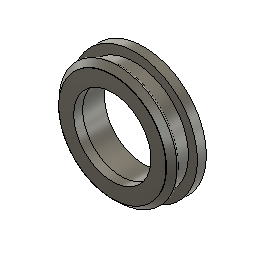
MT2 to 25mm hole sleeve v1 (Autodesk Fusion 360 design; units mm, degrees)
Autodesk Fusion 360 part; units mm, degrees
sketch "Sketch1" plane through (0, 0, 0) normal (0, 0, 1) x (1, 0, 0)
  circle A0 centre (0, 0) radius 8.75
  circle A1 centre (0, 0) radius 12
  circle A2 centre (0, 0) radius 14
  circle A3 centre (0, 0) radius 6
  circle A4 centre (0, 0) radius 2.5
  dimension "d1" = 17.5
  dimension "d2" = 24
  dimension "d3" = 28
  dimension "d8" = 12
  dimension "d11" = 5
  constraint coincident A0.centre A1.centre
  constraint concentric A0 A1
  measures "d1" diameter of A0
  measures "d2" diameter of A1
  measures "d3" diameter of A2
  measures "d8" diameter of A3
  measures "d11" diameter of A4
extrude "Extrude1" add sketch "Sketch1" along normal blind 2 contours A2
extrude "Extrude2" add sketch "Sketch1" along normal blind 5 contours A0 | A1
extrude "Extrude3" cut sketch "Sketch1" along normal blind 5 draft -1.42 contours A0 | A3
sketch "Sketch2" plane through (0, 0, 5) normal (0, 0, 1) x (1, 0, 0)
  circle A0 centre (0, 0) radius 8.6261
  circle A1 centre (0, 0) radius 12
  circle A2 centre (0, 0) radius 8.6261
  circle A3 centre (0, 0) radius 12
  circle A4 centre (0, 0) radius 14
  dimension "d12" = 28
  constraint coincident A0.centre A1.centre
  measures "d12" diameter of A4
extrude "Extrude4" add sketch "Sketch2" along normal blind 2 contours A1 A3
sketch "Sketch3" plane through (0, 0, 0) normal (1, 0, 0) x (0, 0, -1)
  line L0 (-5.3, 12) -> (-5.3, 13)
  line L1 (-5.7268, 13.1768) -> (-6.9036, 12)
  line L2 (-6.9036, 12) -> (-5.3, 12)
  arc A0 (-5.3, 13) -> (-5.7268, 13.1768) centre (-5.55, 13) ccw
  line L3 (-7, 12) -> (-7, -12)
  line L4 (-2, -12) -> (-2, 12)
  line L5 (-5.3, 13) -> (-5, 12)
  line L6 (-5, 12) -> (-5.3, 12)
  dimension "d15" = 0.25
  dimension "d17" = 1
  dimension "d18" = 1.7
  constraint vertical L0
  constraint perpendicular L0 L2
  constraint tangent L0 A0
  constraint tangent L1 A0
  measures "d15" radius of A0
  measures "d17" distance of L2 A0.centre
  measures "d18" distance of L0.start L3.start
revolve "Revolve1" add sketch "Sketch3" angle 360 about axis through (0, 0, 1.75) along (0, 0, 1)
